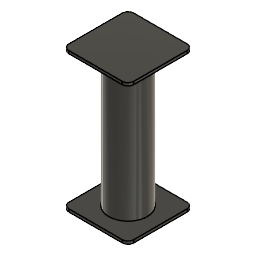
RobotPodium (Autodesk Fusion 360 design; units mm, degrees)
part number: 2026-08-19-14-21-33-033
Autodesk Fusion 360 part; units mm, degrees
sketch "Sketch1" plane through (0, 0, 0) normal (0, 0, 1) x (1, 0, 0)
  line L0 (225, 225) -> (-225, 225)
  line L1 (-225, 225) -> (-225, -225)
  line L2 (-225, -225) -> (225, -225)
  line L3 (225, -225) -> (225, 225)
  line L4 (225, 225) -> (-225, -225) construction
  line L5 (-225, 225) -> (225, -225) construction
  circle A0 centre (0, 0) radius 133.4
  dimension "d1" = 450
  dimension "d2" = 450
  dimension "d3" = 266.8
  constraint horizontal L0
  constraint perpendicular L0 L1
  constraint parallel L0 L2
  constraint parallel L1 L3
  constraint coincident L4 A0.centre
  constraint coincident L5 A0.centre
  constraint coincident A0.centre origin
  measures "d1" distance of L1.end L2.end
  measures "d2" distance of L0.end L1.end
  measures "d3" diameter of A0
extrude "Extrude1" add sketch "Sketch1" along normal blind 20
extrude "Extrude2" add sketch "Sketch1" along normal blind 970 contours A0
sketch "Sketch2" plane through (0, 0, 970) normal (0, 0, 1) x (-1, 0, 0)
  circle A0 centre (0, 0) radius 133.4
  line L0 (225, 225) -> (-225, 225)
  line L1 (-225, 225) -> (-225, -225)
  line L2 (-225, -225) -> (225, -225)
  line L3 (225, -225) -> (225, 225)
  line L4 (225, 225) -> (-225, -225) construction
  line L5 (-225, 225) -> (225, -225) construction
  dimension "d8" = 450
  dimension "d9" = 450
  constraint horizontal L0
  constraint perpendicular L0 L1
  constraint parallel L0 L2
  constraint parallel L1 L3
  constraint coincident L4 A0.centre
  constraint coincident L5 A0.centre
  constraint coincident A0.centre origin
  measures "d8" distance of L1.end L2.end
  measures "d9" distance of L0.end L1.end
extrude "Extrude3" add sketch "Sketch2" against normal blind 20
fillet "Fillet1" radius 40 8 edges at (225, 225, 960) (225, -225, 960) (-225, -225, 960) (-225, 225, 960) (-225, 225, 10) (-225, -225, 10) (225, 225, 10) (225, -225, 10)
